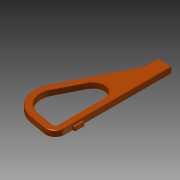
# Autodesk Inventor part: Agarre tijeras (mitad 1)
Saved by Autodesk Inventor 2014 (Build 180170000, 170)
## iProperties
Created: 2016-10-12
Part Number: Agarre tijeras (mitad 1)
Material: Generic
Document SubType Name: Modeling
Designer: Rubén
Density: 1 g/cm^3
Appearance: Smooth - Light Orange
Author: Rubén
Autodesk Inventor part; units mm, degrees
ref_plane "YZ Plane" through (0, 0, 0) normal (1, 0, 0) x (0, 1, 0)
ref_plane "XZ Plane" through (0, 0, 0) normal (0, 1, 0) x (-1, 0, 0)
ref_plane "XY Plane" through (0, 0, 0) normal (0, 0, 1) x (1, 0, 0)
sketch "Sketch1" plane through (0, 0, 0) normal (0, 1, 0) x (-1, 0, 0)
  line L0 (0, 0) -> (0, 56.5412)
  line L1 (5.8682, 61.4653) -> (14.7704, 59.8956)
  line L2 (24.4547, 40.4718) -> (8.4899, 9.1391)
  line L3 (7.4, 4.5992) -> (7.4, 0)
  line L4 (7.4, 0) -> (0, 0)
  line L5 (3.5, 56.5412) -> (3.5, 32.047)
  line L6 (14.846, 29.3231) -> (21.3362, 42.0608)
  line L7 (14.1626, 56.4488) -> (5.2605, 58.0184)
  arc A0 (3.5, 32.047) -> (14.846, 29.3231) centre (9.5, 32.047) ccw
  arc A1 (5.2605, 58.0184) -> (3.5, 56.5412) centre (5, 56.5412) ccw
  arc A2 (5.8682, 61.4653) -> (0, 56.5412) centre (5, 56.5412) ccw
  arc A3 (21.3362, 42.0608) -> (14.1626, 56.4488) centre (12.4261, 46.6007) ccw
  arc A4 (24.4547, 40.4718) -> (14.7704, 59.8956) centre (12.4261, 46.6007) ccw
  arc A5 (8.4899, 9.1391) -> (7.4, 4.5992) centre (17.4, 4.5992) ccw
  point P0 (0, 62.5)
  point P1 (7.4, 7)
  dimension "d0" = 7.4
  dimension "d5" = 27
  dimension "d6" = 80
  dimension "d7" = 7
  dimension "d8" = 6
  dimension "d9" = 1.5
  dimension "d10" = 62.5
  dimension "d12" = 3.5
  dimension "d13" = 10
  dimension "d15" = 10
  constraints: 16 end point, 12 point on circle, 12 tangent, 6 centre point, 4 point on line, 3 parallel, 2 coincident, 2 perpendicular, 1 vertical
  measures "d0" distance of L3.end L0.start
  measures "d5" angle of L0 L2
  measures "d6" angle of L0 L1
  measures "d7" distance of point (7.4, 7) L3.end
  measures "d8" radius of A0
  measures "d9" radius of A1
  measures "d10" distance of L0.start point (0, 62.5)
  measures "d12" distance between parallel lines of L5 L0
  measures "d13" radius of A3
  measures "d15" radius of A5
extrude "Extrusion1" add sketch "Sketch1" along normal blind 3
fillet "Fillet1" radius 0.5 13 edges at (-3.5, 3, 44.2941) (-4.0358, 3, 57.6903) (-9.7116, 3, 57.2336) (-21.3755, 3, 51.0627) (-18.0911, 3, 35.6919) (-8.0993, 3, 26.2128) (-1.7861, 3, 60.3715) (-10.3193, 3, 60.6804) (-24.5078, 3, 52.6243) (-16.4723, 3, 24.8055) (-7.6763, 3, 6.9337) (-7.4, 3, 2.2996) (0, 3, 28.2706)
sketch "Sketch2" plane through (0, 0, 0) normal (0, -1, 0) x (1, 0, 0)
  line L0 (0, 0) -> (0, 56.5412) projected
  line L1 (-7.4, 0) -> (0, 0) projected
  line L2 (0, 52.2) -> (1.25, 52.2)
  line L3 (1.25, 52.2) -> (1.25, 47)
  line L4 (1.25, 47) -> (0, 47)
  dimension "d19" = 1.25
  dimension "d20" = 5.2
  dimension "d21" = 47
  constraints: 6 end point, 2 perpendicular, 2 point on line, 1 parallel
  measures "d19" distance of L3.end L4.end
  measures "d20" distance of L2.end L3.end
  measures "d21" distance between parallel lines of L4 L1
extrude "Extrusion2" add sketch "Sketch2" against normal blind 2
fillet "Fillet2" radius 0.5 8 edges at (1.25, 2, 49.6) (1.25, 1, 52.2) (0.625, 2, 52.2) (0.625, 2, 47) (1.25, 1, 47) (0, 1, 52.2) (0, 2, 49.6) (0, 1, 47)
body "Solid1"
